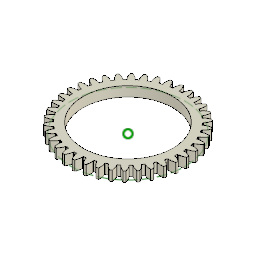
gear-wheel v2 (Autodesk Fusion 360 design; units mm, degrees)
description: Spur Gear; Module: 0.300000; Num Teeth: 38; Pressure Angle: 20.000000; Backlash: 0.00 mm
Autodesk Fusion 360 part; units mm, degrees
sketch "スケッチ1" plane through (0, 0, 0) normal (0, 0, 1) x (1, 0, 0) in component "Spur Gear (38 teeth)"
  circle A0 centre (0, 0) radius 5.2892
  circle A1 centre (0, 0) radius 4.5
extrude "押し出し1" add sketch "スケッチ1" along normal blind 1 in component "Spur Gear (38 teeth)"
sketch "スケッチ2" plane through (0, 0, 0) normal (0, 0, 1) x (1, 0, 0) in component "Spur Gear (38 teeth)"
  spline S0 degree 5 poles (5.3478, -0.3011) (5.3496, -0.3012) (5.3533, -0.3013) (5.3589, -0.3014) (5.3663, -0.3014) (5.3756, -0.301) (5.3849, -0.3004) (5.3942, -0.2996) (5.4035, -0.2988) (5.4128, -0.2979) (5.4221, -0.2969) (5.4314, -0.2959) (5.4408, -0.2948) (5.4501, -0.2935) (5.4594, -0.2922) (5.4687, -0.2907) (5.4781, -0.2892) (5.4874, -0.2876) (5.4967, -0.2859) (5.5061, -0.2842) (5.5154, -0.2824) (5.5247, -0.2805) (5.5341, -0.2786) (5.5434, -0.2766) (5.5527, -0.2745) (5.5621, -0.2723) (5.5714, -0.2701) (5.5807, -0.2679) (5.5901, -0.2656) (5.5994, -0.2632) (5.6087, -0.2607) (5.6181, -0.2582) (5.6274, -0.2557) (5.6367, -0.2531) (5.6461, -0.2504) (5.6554, -0.2477) (5.6647, -0.245) (5.674, -0.2421) (5.6834, -0.2393) (5.6927, -0.2363) (5.702, -0.2334) (5.7113, -0.2303) (5.7207, -0.2273) (5.73, -0.2241) (5.7393, -0.221) (5.7486, -0.2177) (5.7579, -0.2145) (5.7672, -0.2111) (5.7765, -0.2078) (5.7858, -0.2044) (5.7951, -0.2009) (5.8044, -0.1974) (5.8137, -0.1938) (5.823, -0.1902) (5.8323, -0.1866) (5.8416, -0.1829) (5.8509, -0.1792) (5.8602, -0.1754) (5.8694, -0.1716) (5.8787, -0.1677) (5.888, -0.1638) (5.8972, -0.1598) (5.9065, -0.1558) (5.9158, -0.1518) (5.925, -0.1477) (5.9343, -0.1436) (5.9435, -0.1394) (5.9528, -0.1352) (5.962, -0.131) (5.9712, -0.1267) (5.9805, -0.1223) (5.9879, -0.1188) (5.9934, -0.1162) (5.9971, -0.1144) (5.9989, -0.1135) knots 0 0 0 0 0 0 0.01428571 0.02857143 0.04285714 0.05714286 0.07142857 0.08571429 0.1 0.11428571 0.12857143 0.14285714 0.15714286 0.17142857 0.18571429 0.2 0.21428571 0.22857143 0.24285714 0.25714286 0.27142857 0.28571429 0.3 0.31428571 0.32857143 0.34285714 0.35714286 0.37142857 0.38571429 0.4 0.41428571 0.42857143 0.44285714 0.45714286 0.47142857 0.48571429 0.5 0.51428571 0.52857143 0.54285714 0.55714286 0.57142857 0.58571429 0.6 0.61428571 0.62857143 0.64285714 0.65714286 0.67142857 0.68571429 0.7 0.71428571 0.72857143 0.74285714 0.75714286 0.77142857 0.78571429 0.8 0.81428571 0.82857143 0.84285714 0.85714286 0.87142857 0.88571429 0.9 0.91428571 0.92857143 0.94285714 0.95714286 0.97142857 0.98571429 1 1 1 1 1 1
  spline S1 degree 5 poles (5.3478, 0.3011) (5.3496, 0.3012) (5.3533, 0.3013) (5.3589, 0.3014) (5.3663, 0.3014) (5.3756, 0.301) (5.3849, 0.3004) (5.3942, 0.2996) (5.4035, 0.2988) (5.4128, 0.2979) (5.4221, 0.2969) (5.4314, 0.2959) (5.4408, 0.2948) (5.4501, 0.2935) (5.4594, 0.2922) (5.4687, 0.2907) (5.4781, 0.2892) (5.4874, 0.2876) (5.4967, 0.2859) (5.5061, 0.2842) (5.5154, 0.2824) (5.5247, 0.2805) (5.5341, 0.2786) (5.5434, 0.2766) (5.5527, 0.2745) (5.5621, 0.2723) (5.5714, 0.2701) (5.5807, 0.2679) (5.5901, 0.2656) (5.5994, 0.2632) (5.6087, 0.2607) (5.6181, 0.2582) (5.6274, 0.2557) (5.6367, 0.2531) (5.6461, 0.2504) (5.6554, 0.2477) (5.6647, 0.245) (5.674, 0.2421) (5.6834, 0.2393) (5.6927, 0.2363) (5.702, 0.2334) (5.7113, 0.2303) (5.7207, 0.2273) (5.73, 0.2241) (5.7393, 0.221) (5.7486, 0.2177) (5.7579, 0.2145) (5.7672, 0.2111) (5.7765, 0.2078) (5.7858, 0.2044) (5.7951, 0.2009) (5.8044, 0.1974) (5.8137, 0.1938) (5.823, 0.1902) (5.8323, 0.1866) (5.8416, 0.1829) (5.8509, 0.1792) (5.8602, 0.1754) (5.8694, 0.1716) (5.8787, 0.1677) (5.888, 0.1638) (5.8972, 0.1598) (5.9065, 0.1558) (5.9158, 0.1518) (5.925, 0.1477) (5.9343, 0.1436) (5.9435, 0.1394) (5.9528, 0.1352) (5.962, 0.131) (5.9712, 0.1267) (5.9805, 0.1223) (5.9879, 0.1188) (5.9934, 0.1162) (5.9971, 0.1144) (5.9989, 0.1135) knots 0 0 0 0 0 0 0.01428571 0.02857143 0.04285714 0.05714286 0.07142857 0.08571429 0.1 0.11428571 0.12857143 0.14285714 0.15714286 0.17142857 0.18571429 0.2 0.21428571 0.22857143 0.24285714 0.25714286 0.27142857 0.28571429 0.3 0.31428571 0.32857143 0.34285714 0.35714286 0.37142857 0.38571429 0.4 0.41428571 0.42857143 0.44285714 0.45714286 0.47142857 0.48571429 0.5 0.51428571 0.52857143 0.54285714 0.55714286 0.57142857 0.58571429 0.6 0.61428571 0.62857143 0.64285714 0.65714286 0.67142857 0.68571429 0.7 0.71428571 0.72857143 0.74285714 0.75714286 0.77142857 0.78571429 0.8 0.81428571 0.82857143 0.84285714 0.85714286 0.87142857 0.88571429 0.9 0.91428571 0.92857143 0.94285714 0.95714286 0.97142857 0.98571429 1 1 1 1 1 1
  arc A0 (5.9989, -0.1135) -> (5.9989, 0.1135) centre (0, 0) ccw
  line L0 (5.2709, -0.2973) -> (5.3478, -0.3011)
  line L1 (5.2709, 0.2973) -> (5.3478, 0.3011)
  line L2 (5.2709, -0.2973) -> (5.2709, 0.2973)
extrude "押し出し2" add sketch "スケッチ2" along normal blind 1 in component "Spur Gear (38 teeth)"
pattern_circular "C パターン1" count 38 over 360 about axis through (0, 0, 0) along (0, 0, 1) of "押し出し2" in component "Spur Gear (38 teeth)"
sketch "スケッチ3" plane through (0, 0, 0) normal (0, 0, 1) x (1, 0, 0) in component "Spur Gear (38 teeth)"
  circle A0 centre (0, 0) radius 5.7 construction
component "Spur Gear (38 teeth)" placed x (1, 0, 0) y (0, 1, 0) z (0, 0, 1) at (0, 0, 3.5)
